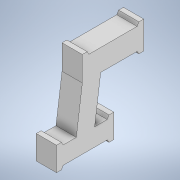
# Autodesk Inventor part: Big Housing
Saved by Autodesk Inventor 2022 (Build 260153000, 153)
## iProperties
Created: 2021-06-03
Part Number: Big Housing
Material: Generic
Document SubType Name: Modeling
Designer: jrcol
Density: 1 g/cm^3
Appearance: Default
Author: jrcol
Autodesk Inventor part; units mm, degrees
ref_plane "YZ Plane" through (0, 0, 0) normal (1, 0, 0) x (0, 1, 0)
ref_plane "XZ Plane" through (0, 0, 0) normal (0, 1, 0) x (-1, 0, 0)
ref_plane "XY Plane" through (0, 0, 0) normal (0, 0, 1) x (1, 0, 0)
sketch "Sketch3" plane through (0, 0, 0) normal (1, 0, 0) x (0, 1, 0)
  line L0 (0, 0) -> (48.9982, 0)
  line L1 (48.9982, -15.0415) -> (48.9982, -124.2618)
  line L2 (48.9982, -139.3032) -> (0.0211, -139.3032)
  line L3 (0.0211, -124.2618) -> (0.0211, -41.5471)
  line L4 (0, 0) -> (-99.9892, 13.7012)
  line L5 (-99.9892, -27.843) -> (0.0211, -41.5471)
  line L6 (48.9982, -139.3032) -> (55.9982, -139.3032)
  line L7 (55.9982, -139.3032) -> (55.9982, -128.3032)
  line L8 (55.9982, -128.3032) -> (48.9982, -124.2618)
  line L9 (48.9982, 0) -> (55.9982, 0)
  line L10 (55.9982, 0) -> (55.9982, -11)
  line L11 (55.9982, -11) -> (48.9982, -15.0415)
  line L12 (0.0211, -139.3032) -> (-6.9789, -139.3032)
  line L13 (-6.9789, -139.3032) -> (-6.9789, -128.3032)
  line L14 (-6.9789, -128.3032) -> (0.0211, -124.2618)
  line L15 (-148.6902, -63.3226) -> (-148.65, -63.3226)
  line L16 (-99.9892, -27.843) -> (-99.9892, -56.4562)
  line L17 (-99.9789, -71.5036) -> (-139.9913, -71.5036)
  line L18 (-139.9892, -56.4622) -> (-139.9892, 43.4549)
  line L19 (-139.9892, 58.4964) -> (-99.9892, 58.4964)
  line L20 (-99.9892, 43.4549) -> (-99.9892, 13.7012)
  line L21 (-99.9789, -71.5036) -> (-92.9789, -71.5036)
  line L22 (-92.9789, -71.5036) -> (-92.9789, -60.5036)
  line L23 (-92.9789, -60.5036) -> (-99.9892, -56.4562)
  line L24 (-139.9913, -71.5036) -> (-146.9913, -71.5036)
  line L25 (-146.9913, -71.5036) -> (-146.9913, -60.5036)
  line L26 (-146.9913, -60.5036) -> (-139.9892, -56.4622)
  line L27 (-139.9892, 58.4964) -> (-146.9892, 58.4964)
  line L28 (-146.9892, 58.4964) -> (-146.9892, 47.4964)
  line L29 (-146.9892, 47.4964) -> (-139.9892, 43.4549)
  line L30 (-99.9892, 58.4964) -> (-92.9892, 58.4964)
  line L31 (-92.9892, 58.4964) -> (-92.9892, 47.4964)
  line L32 (-92.9892, 47.4964) -> (-99.9892, 43.4549)
  dimension "d11" = 120
  dimension "d12" = 7
  dimension "d13" = 11
  dimension "d16" = 130
  dimension "d17" = 40
  dimension "d18" = 7
  dimension "d19" = 11
  dimension "d20" = 120
  dimension "d21" = 120
  constraints: 66 end point, 12 perpendicular, 11 equal length, 7 horizontal, 3 parallel, 3 point on line, 1 vertical
  measures "d11" angle of L1 L11
  measures "d12" distance of L2.start L6.end
  measures "d13" distance of L6.end L7.end
  measures "d16" distance of L17.end L19.start
  measures "d17" distance of L19.start L19.end
  measures "d18" distance of L17.start L21.end
  measures "d19" distance of L21.end L22.end
  measures "d20" angle of L23 L22
  measures "d21" angle of L28 L29
extrude "Extrusion1" add sketch "Sketch3" along normal mid plane 46
body "Solid1"
